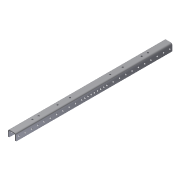
# Autodesk Inventor part: C Channel 2 1764
Saved by Autodesk Inventor 2011 (Build 150239000, 239)
## iProperties
Created: 2009-01-11
Part Number: C Channel 2 1764
Document SubType Name: Modeling
Designer: jrobinson
Density: 1 g/cm^3
Author: jrobinson
Autodesk Inventor part; units mm, degrees
ref_plane "YZ Plane" through (0, 0, 0) normal (1, 0, 0) x (0, 1, 0)
ref_plane "XZ Plane" through (0, 0, 0) normal (0, 1, 0) x (-1, 0, 0)
sketch "Sketch1" plane through (0, 0, 0) normal (0, 0, 1) x (1, 0, 0)
  line L0 (-25.9259, -4.2593) -> (-25.9259, 24.3157)
  line L1 (-25.9259, 24.3157) -> (5.8241, 24.3157)
  line L2 (5.8241, 24.3157) -> (5.8241, -4.2593)
  line L3 (5.8241, -4.2593) -> (2.6491, -4.2593)
  line L4 (2.6491, -4.2593) -> (2.6491, 21.1407)
  line L5 (2.6491, 21.1407) -> (-22.7509, 21.1407)
  line L6 (-22.7509, 21.1407) -> (-22.7509, -4.2593)
  line L7 (-22.7509, -4.2593) -> (-25.9259, -4.2593)
  dimension "d0" = 25.4
  dimension "d1" = 31.75
  dimension "d2" = 3.175
  dimension "d3" = 3.175
  dimension "d4" = 28.575
  dimension "d5" = 0
  constraints: 16 end point, 6 parallel, 1 perpendicular, 1 vertical
  measures "d0" distance between parallel lines of L4 L6
  measures "d1" distance between parallel lines of L0 L2
  measures "d2" distance between parallel lines of L2 L4
  measures "d3" distance between parallel lines of L1 L5
  measures "d4" distance between parallel lines of L1 L3
  measures "d5" distance between parallel lines of L7 L3
extrude "Extrusion1" add sketch "Sketch1" along normal blind 889
fillet "Fillet1" radius 6.35 4 edges at (-22.7509, 21.1407, 444.5) (-25.9259, 24.3157, 444.5) (5.8241, 24.3157, 444.5) (2.6491, 21.1407, 444.5)
fillet "Fillet2" radius 3.175 4 edges at (4.2366, -4.2593, 889) (-24.3384, -4.2593, 889) (-24.3384, -4.2593, 0) (4.2366, -4.2593, 0)
sketch "Sketch2" plane through (-25.9259, 17.9657, 0) normal (-1, 0, 0) x (0, 0, 1)
  line L0 (3.175, -22.225) -> (885.825, -22.225) projected
  line L1 (0, -19.05) -> (0, 0) projected
  circle A0 centre (12.7, -9.525) radius 3.175
  dimension "d10" = 6.35
  dimension "d11" = 12.7
  dimension "d12" = 12.7
  constraints: 1 centre point
  measures "d10" diameter of A0
  measures "d11" distance from line of L0 A0.centre
  measures "d12" distance from line of L1 A0.centre
extrude "Extrusion2" cut sketch "Sketch2" against normal through all
pattern_linear "Rectangular Pattern1" count 35 spacing 25.4 along (0, 0, 1) of "Extrusion2"
ref_plane "Work Plane2" through (67.878, 24.3157, 444.5) normal (0, 0, -1) x (-1, 0, 0)
sketch "Sketch6" plane through (5.8241, 17.9657, 889) normal (1, 0, 0) x (0, 0, -1)
  circle A0 centre (698.5, -9.525) radius 3.175 projected
  circle A1 centre (723.9, -9.525) radius 3.175 projected
  circle A2 centre (749.3, -9.525) radius 3.175 projected
  circle A3 centre (774.7, -9.525) radius 3.175 projected
  circle A4 centre (800.1, -9.525) radius 3.175 projected
  circle A5 centre (825.5, -9.525) radius 3.175 projected
  circle A6 centre (850.9, -9.525) radius 3.175 projected
  circle A7 centre (876.3, -9.525) radius 3.175 projected
  line L0 (976.9561, 155.027) -> (631.825, 155.027)
  line L1 (631.825, 155.027) -> (631.825, -109.3216)
  line L2 (631.825, -109.3216) -> (976.9561, -109.3216)
  line L3 (976.9561, -109.3216) -> (976.9561, 155.027)
  line L4 (0, 0) -> (0, -19.05) projected
  dimension "d54" = 631.825
  constraints: 8 end point, 2 parallel, 1 horizontal, 1 perpendicular
  measures "d54" distance between parallel lines of L1 L4
extrude "Extrusion5" cut sketch "Sketch6" against normal through all
sketch "Sketch8" plane through (-19.5759, 24.3157, 889) normal (0, 1, 0) x (1, 0, 0)
  line L0 (19.05, 631.825) -> (0, 631.825) projected
  line L1 (0, 0) -> (19.05, 0) projected
  circle A0 centre (9.525, 82.55) radius 3.175
  circle A1 centre (9.525, 107.95) radius 3.175
  circle A2 centre (9.525, 184.15) radius 3.175
  circle A3 centre (9.525, 234.95) radius 3.175
  circle A4 centre (9.525, 549.275) radius 3.175
  circle A5 centre (9.525, 396.875) radius 3.175
  circle A6 centre (9.525, 523.875) radius 3.175
  circle A7 centre (9.525, 447.675) radius 3.175
  point P0 (19.5759, 889)
  point P1 (9.525, 0)
  dimension "d43" = 6.35
  dimension "d44" = 82.55
  dimension "d45" = 25.4
  dimension "d46" = 76.2
  dimension "d47" = 50.8
  dimension "d48" = 82.55
  dimension "d49" = 25.4
  dimension "d50" = 76.2
  dimension "d51" = 50.8
  constraints: 8 centre point, 8 vertical alignment, 7 equal radius, 1 midpoint
  measures "d43" diameter of A0
  measures "d44" distance from line of A0.centre L1
  measures "d45" distance of A1.centre A0.centre
  measures "d46" distance of A2.centre A1.centre
  measures "d47" distance of A3.centre A2.centre
  measures "d48" distance from line of L0 A4.centre
  measures "d49" distance of A6.centre A4.centre
  measures "d50" distance of A7.centre A6.centre
  measures "d51" distance of A5.centre A7.centre
extrude "Extrusion7" cut sketch "Sketch8" along normal through all both and the other way through all
sketch "Sketch9" plane through (5.8241, -4.2593, 257.175) normal (0, -1, 0) x (1, 0, 0)
  line L0 (-3.175, 0) -> (0, 0) projected
  line L1 (0, 0) -> (0, 628.65) projected
  line L2 (-3.175, 628.65) -> (0, 628.65) projected
  line L3 (-3.175, 0) -> (-3.175, 628.65) projected
  line L4 (-31.75, 0) -> (-28.575, 0) projected
  line L5 (-28.575, 0) -> (-28.575, 628.65) projected
  line L6 (-31.75, 628.65) -> (-28.575, 628.65) projected
  line L7 (-31.75, 0) -> (-31.75, 628.65) projected
  point P0 (-5.8241, -257.175)
sketch "Sketch10" plane through (-25.9259, -1.0843, 889) normal (-1, 0, 0) x (0, 0, 1)
  circle A0 centre (-304.8, 9.525) radius 3.175 projected
  circle A1 centre (-330.2, 9.525) radius 3.175 projected
  circle A2 centre (-304.8, 9.525) radius 3.175
  circle A3 centre (-330.2, 9.525) radius 3.175
  circle A4 centre (-279.4, 9.525) radius 3.175
  circle A5 centre (-355.6, 9.525) radius 3.175
  point P0 (-889, 1.0843)
  dimension "d55" = 6.35
  dimension "d56" = 6.35
  dimension "d57" = 25.4
  dimension "d58" = 50.8
  constraints: 4 centre point, 2 coincident, 2 concentric
  measures "d55" diameter of A4
  measures "d56" diameter of A5
  measures "d57" distance of A0.centre A4.centre
  measures "d58" distance of A5.centre A0.centre
extrude "Extrusion8" cut sketch "Sketch10" against normal blind 38.1
sketch "Sketch11" plane through (0, 0, 889) normal (0, 0, 1) x (1, 0, 0)
  line L0 (-22.7509, -1.0843) -> (-25.9259, -1.0843) projected
  line L1 (-22.7509, 14.7907) -> (-22.7509, -1.0843) projected
  arc A0 (-16.4009, 21.1407) -> (-22.7509, 14.7907) centre (-16.4009, 14.7907) ccw projected
  line L2 (-3.7009, 21.1407) -> (-16.4009, 21.1407) projected
  arc A1 (2.6491, 14.7907) -> (-3.7009, 21.1407) centre (-3.7009, 14.7907) ccw projected
  line L3 (2.6491, -1.0843) -> (2.6491, 14.7907) projected
  line L4 (5.8241, -1.0843) -> (2.6491, -1.0843) projected
  line L5 (5.8241, 17.9657) -> (5.8241, -1.0843) projected
  arc A2 (5.8241, 17.9657) -> (-0.5259, 24.3157) centre (-0.5259, 17.9657) ccw projected
  line L6 (-19.5759, 24.3157) -> (-0.5259, 24.3157) projected
  arc A3 (-19.5759, 24.3157) -> (-25.9259, 17.9657) centre (-19.5759, 17.9657) ccw projected
  line L7 (-25.9259, -1.0843) -> (-25.9259, 17.9657) projected
  line L8 (-25.9259, -4.2593) -> (-22.7509, -4.2593) projected
  line L9 (2.6491, -4.2593) -> (5.8241, -4.2593) projected
  line L10 (-90.542, -90.1503) -> (-1.8937, -1.502)
  line L11 (-25.9259, 17.9657) -> (-25.9259, -25.5343)
  line L12 (4.9313, -8.327) -> (-83.0857, -96.3441)
  line L13 (-25.9259, 17.9657) -> (-25.9259, -39.1843)
  line L14 (-19.5759, 24.3157) -> (-31.8681, 24.3157)
  line L15 (-25.9259, 24.3157) -> (-25.9259, -39.1843)
  point P0 (0, 0)
  dimension "d61" = 49.85
  dimension "d62" = 63.5
  constraints: 12 end point, 3 perpendicular, 3 point on line, 3 tangent, 1 collinear, 1 point on circle, 6 other
  measures "d61" distance from line of L11.end L6
  measures "d62" distance from line of L13.end L6
body "Solid1"
